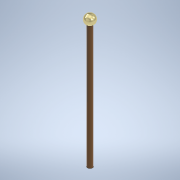
# Autodesk Inventor part: FlagPole
Saved by Autodesk Inventor 2021 (Build 250183000, 183)
## iProperties
Created: 2021-03-22
Part Number: FlagPole
Material: Générique
Document SubType Name: Modeling
Designer: turnb
Density: 1 g/cm^3
Appearance: Par défaut
Author: turnb
Autodesk Inventor part; units mm, degrees
ref_plane "YZ Plane" through (0, 0, 0) normal (1, 0, 0) x (0, 1, 0)
ref_plane "XZ Plane" through (0, 0, 0) normal (0, 1, 0) x (-1, 0, 0)
ref_plane "XY Plane" through (0, 0, 0) normal (0, 0, 1) x (1, 0, 0)
sketch "Esquisse1" plane through (0, 0, 0) normal (0, 0, 1) x (1, 0, 0)
  line L0 (-7.5, -232.9053) -> (7.5, -232.9053)
  line L1 (7.5, -232.9053) -> (7.5, 138.4158)
  line L2 (-7.5, 138.4158) -> (-7.5, -232.9053)
  line L3 (-7.5, -232.9053) -> (4.4139, 137.0703) construction
  line L4 (7.5, -232.9053) -> (-4.4139, 137.0703) construction
  circle A0 centre (0, 151.4062) radius 15
  line L5 (0, -232.9053) -> (0, 166.4062)
  point P0 (0, 0)
  dimension "d1" = 30
  constraints: 12 end point, 5 point on circle, 2 parallel, 2 point on line, 1 centre point, 1 horizontal, 1 midpoint, 1 perpendicular
  measures "d1" diameter of A0
revolve "Révolution1" add sketch "Esquisse1" angle 360 about axis through (0, -232.9053, 0) along (0, 1, 0) picked at (3.1174, 155.3154) contours L5 A0 L1 L0 | L5 A0
sketch "Esquisse2" plane through (0, 0, 0) normal (1, 0, 0) x (0, 1, 0)
  line L0 (138.4158, 7.5) -> (138.4158, -7.5) projected
  line L1 (138.4158, -7.5) -> (-232.9053, -7.5) projected
  line L2 (138.4158, 7.5) -> (-61.5842, 7.5)
  line L3 (-61.5842, 7.5) -> (-61.5842, -7.5)
  line L4 (-61.5842, -7.5) -> (138.4158, -7.5)
  line L5 (138.4158, -7.5) -> (138.4158, 7.5)
  point P0 (0, 0)
  dimension "d3" = 200
  constraints: 8 end point, 2 parallel, 1 horizontal, 1 perpendicular, 1 point on line
  measures "d3" distance of L4.end L3.end
extrude "Extrusion1" add sketch "Esquisse2" along normal blind 0.1
